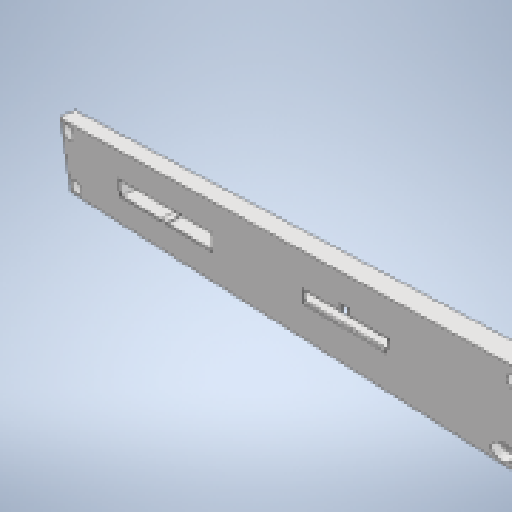
# Autodesk Inventor part: FrontPlate
Saved by Autodesk Inventor 2025.2 (Build 292293000, 293)
## iProperties
Created: 2025-08-10
Part Number: FrontPlate
Material: Generic
Document SubType Name: Modeling
Designer: hofma
Density: 1 g/cm^3
Appearance: Default
Author: hofma
Autodesk Inventor part; units mm, degrees
note: some values were not read from the file. Chosen so that the rebuilt part matches the saved one: direction of "Hole1".
ref_plane "YZ Plane" through (0, 0, 0) normal (1, 0, 0) x (0, 1, 0)
ref_plane "XZ Plane" through (0, 0, 0) normal (0, 1, 0) x (-1, 0, 0)
ref_plane "XY Plane" through (0, 0, 0) normal (0, 0, 1) x (1, 0, 0)
sketch "Sketch1" plane through (0, 0, 0) normal (0, 0, 1) x (1, 0, 0)
  line L0 (-125, 20) -> (125, 20)
  line L1 (125, 20) -> (125, -20)
  line L2 (125, -20) -> (-125, -20)
  line L3 (-125, -20) -> (-125, 20)
  line L4 (-125, 20) -> (125, -20) construction
  line L5 (125, 20) -> (-125, -20) construction
  point P0 (0, 0)
  dimension "d0" = 250
  dimension "d1" = 40
  constraints: 12 end point, 2 midpoint, 2 parallel, 1 horizontal, 1 perpendicular
  measures "d0" distance of L0.start L0.end
  measures "d1" distance of L2.end L0.start
extrude "Extrusion1" add sketch "Sketch1" along normal blind 10
sketch "Sketch2" plane through (0, 0, 10) normal (0, 0, 1) x (1, 0, 0)
  line L0 (30.75, 2.75) -> (69.25, 2.75)
  line L1 (69.25, 2.75) -> (69.25, -2.75)
  line L2 (69.25, -2.75) -> (30.75, -2.75)
  line L3 (30.75, -2.75) -> (30.75, 2.75)
  line L4 (-80.6, 4.125) -> (-19.4, 4.125)
  line L5 (-19.4, 4.125) -> (-19.4, -4.125)
  line L6 (-19.4, -4.125) -> (-80.6, -4.125)
  line L7 (-80.6, -4.125) -> (-80.6, 4.125)
  line L8 (-125, 20) -> (-125, -20) projected
  line L9 (-125, 0) -> (125, 0) construction
  line L10 (125, -20) -> (125, 20) projected
  line L11 (-125, 20) -> (0, 20) construction
  line L12 (125, 20) -> (-125, 20) construction
  line L13 (0, 20) -> (125, 20) construction
  line L14 (48.7, 2.75) -> (51.3, 2.75)
  line L15 (51.3, 2.75) -> (51.3, 5.95)
  line L16 (51.3, 5.95) -> (48.7, 5.95)
  line L17 (48.7, 5.95) -> (48.7, 2.75)
  point P0 (0, 0)
  point P1 (-62.5, 20)
  point P2 (-50, 4.125)
  point P3 (62.5, 20)
  point P4 (50, 2.75)
  point P5 (-19.4, 0)
  point P6 (30.75, 0)
  point P7 (50, 5.95)
  point P8 (0, 0)
  dimension "d5" = 61.2
  dimension "d6" = 8.25
  dimension "d7" = 0
  dimension "d8" = 38.5
  dimension "d9" = 5.5
  dimension "d10" = 2.6
  dimension "d12" = 8.7
  dimension "d35" = 50
  dimension "d52" = 50
  constraints: 30 end point, 11 midpoint, 6 parallel, 4 horizontal, 3 perpendicular, 3 point on line, 1 collinear, 1 vertical alignment
  measures "d5" distance of L4.start L4.end
  measures "d6" distance between parallel lines of L6 L4
  measures "d7" distance from line of point (0, 0) L9
  measures "d8" distance between parallel lines of L1 L3
  measures "d9" distance between parallel lines of L2 L0
  measures "d10" distance of L15.end L16.end
  measures "d12" distance between parallel lines of L16 L2
  measures "d35" horizontal distance of point (50, 5.95) point (0, 0)
  measures "d52" horizontal distance of point (0, 0) point (-50, 4.125)
extrude "Extrusion2" cut sketch "Sketch2" against normal through all
sketch "Sketch3" plane through (-80.6, -4.125, 10) normal (0, 1, 0) x (1, 0, 0)
  line L0 (0, 0) -> (0, 10) projected
  line L1 (61.2, 0) -> (61.2, 10) projected
  line L2 (-44.4, 0) -> (205.6, 0) projected
  line L3 (28.6, 0) -> (32.6, 0)
  line L4 (32.6, 0) -> (32.6, 7.6)
  line L5 (32.6, 7.6) -> (28.6, 7.6)
  line L6 (28.6, 7.6) -> (28.6, 0)
  line L7 (0, 10) -> (61.2, 10) construction
  line L8 (-44.4, 10) -> (205.6, 10) projected
  point P0 (80.6, 10)
  point P1 (30.6, 10)
  point P2 (30.6, 7.6)
  dimension "d15" = 4
  dimension "d16" = 7.6
  constraints: 10 end point, 2 midpoint, 2 parallel, 1 collinear, 1 horizontal, 1 perpendicular, 1 point on line, 1 vertical alignment
  measures "d15" distance of L4.end L5.end
  measures "d16" distance of L5.end L3.start
extrude "Extrusion3" add sketch "Sketch3" along normal blind 0.8 contours L6 L5 L4 L2
sketch "Sketch4" plane through (0, 0, 0) normal (0, 0, -1) x (-1, 0, 0)
  line L0 (-90, 5.95) -> (-10, 5.95)
  line L1 (-10, 5.95) -> (-10, -7.05)
  line L2 (-10, -7.05) -> (-90, -7.05)
  line L3 (-90, -7.05) -> (-90, 5.95)
  line L4 (-51.3, 5.95) -> (-48.7, 5.95) projected
  point P0 (0, 0)
  point P1 (-50, 5.95)
  point P2 (-50, 5.95)
  dimension "d19" = 80
  dimension "d20" = 13
  constraints: 8 end point, 3 midpoint, 2 parallel, 1 coincident, 1 horizontal, 1 perpendicular
  measures "d19" distance of L0.start L0.end
  measures "d20" distance of L2.end L0.start
extrude "Extrusion4" cut sketch "Sketch4" against normal blind 8
sketch "Sketch6" plane through (10, -7.05, 0) normal (0, 1, 0) x (1, 0, 0)
  line L0 (0, 0) -> (80, 0) projected
  line L1 (40, 0) -> (40, -18.0436) construction
  line L2 (-135, -10) -> (115, -10) projected
  line L3 (67.5, 0) -> (74.5, 0)
  line L4 (74.5, 0) -> (74.5, -10)
  line L5 (74.5, -10) -> (67.5, -10)
  line L6 (67.5, -10) -> (67.5, 0)
  line L7 (-135, 0) -> (115, 0) projected
  line L8 (5.5, -10) -> (12.5, -10)
  line L9 (12.5, -10) -> (12.5, 0)
  line L10 (12.5, 0) -> (5.5, 0)
  line L11 (5.5, 0) -> (5.5, -10)
  point P0 (-10, 0)
  point P1 (9, -10)
  point P2 (71, -10)
  dimension "d28" = 62
  dimension "d29" = 7
  constraints: 18 end point, 4 parallel, 3 midpoint, 3 point on line, 2 horizontal, 2 perpendicular, 1 vertical, 4 other
  measures "d28" distance of point (9, -10) point (71, -10)
  measures "d29" distance between parallel lines of L6 L4
extrude "Extrusion6" add sketch "Sketch6" along normal blind 3.116 contours L0 L9 L2 L11 | L0 L4 L2 L6
sketch "Sketch7" plane through (0, 0, 0) normal (0, 0, -1) x (-1, 0, 0)
  line L0 (-84.5, -3.934) -> (-77.5, -3.934) projected
  line L1 (-84.5, -7.05) -> (-84.5, -3.934) projected
  line L2 (-77.5, -7.05) -> (-77.5, -3.934) projected
  line L3 (-22.5, -3.934) -> (-15.5, -3.934) projected
  line L4 (-15.5, -7.05) -> (-15.5, -3.934) projected
  line L5 (-22.5, -7.05) -> (-22.5, -3.934) projected
  line L6 (-84.5, -7.05) -> (-90, -7.05) projected
  line L7 (-84.5, -7.05) -> (-77.5, -7.05)
  line L8 (-77.5, -7.05) -> (-77.5, -9.934)
  line L9 (-77.5, -9.934) -> (-84.5, -9.934)
  line L10 (-84.5, -9.934) -> (-84.5, -7.05)
  line L11 (-22.5, -7.05) -> (-77.5, -7.05) projected
  line L12 (-22.5, -7.05) -> (-15.5, -7.05)
  line L13 (-15.5, -7.05) -> (-15.5, -9.934)
  line L14 (-15.5, -9.934) -> (-22.5, -9.934)
  line L15 (-22.5, -9.934) -> (-22.5, -7.05)
  point P0 (0, 0)
  point P1 (-81, -9.934)
  point P2 (-19, -9.934)
  point P3 (-77.5, -5.492)
  point P4 (-77.5, -8.492)
  point P5 (-15.5, -5.492)
  point P6 (-15.5, -8.492)
  dimension "d32" = 6
  constraints: 16 end point, 6 midpoint, 4 parallel, 2 horizontal, 2 perpendicular, 2 vertical alignment, 1 horizontal alignment
  measures "d32" distance between parallel lines of L9 L0
extrude "Extrusion7" add sketch "Sketch7" along normal blind 2
sketch "Sketch8" plane through (0, 0, 10) normal (0, 0, 1) x (1, 0, 0)
  line L0 (125, 20) -> (-125, 20) projected
  line L1 (-125, 20) -> (-125, -20) projected
  line L2 (125, -20) -> (125, 20) projected
  line L3 (-125, -20) -> (125, -20) projected
  point P0 (0, 0)
  point P1 (-117.5, 15)
  point P2 (-117.5, -15)
  point P3 (117.5, 15)
  point P4 (117.5, -15)
  dimension "d36" = 5
  dimension "d37" = 7.5
  dimension "d38" = 7.5
  dimension "d39" = 5
  constraints: 2 horizontal alignment, 2 vertical alignment
  measures "d36" distance from line of point (-117.5, 15) L0
  measures "d37" distance from line of L1 point (-117.5, 15)
  measures "d38" distance from line of L2 point (117.5, 15)
  measures "d39" distance from line of L3 point (-117.5, -15)
hole "Hole1" at (117.5, -15, 10) at (-117.5, 15, 10) at (117.5, 15, 10) at (-117.5, -15, 10) direction (0, 0, -1) diameter 4.2 depth 10 counterbore diameter 8 counterbore depth 4.6 clearance for "Socket Head Cap Screw ISO 4762" size "M4" standard "ISO"
sketch "Sketch9" plane through (10, -3.934, 0) normal (0, 1, 0) x (1, 0, 0)
  circle A0 centre (71.05, -1.5002) radius 1.95 projected
  circle A1 centre (9.05, -1.5002) radius 1.95 projected
  point P0 (-10, 0)
extrude "Extrusion8" cut sketch "Sketch9" against normal blind 6
chamfer "Chamfer1" distance 7 angle 45 1 edges at (50, 5.95, 0)
chamfer "Chamfer2" distance 2 angle 45 2 edges at (-125, 0, 10) (125, 0, 10)
chamfer "Chamfer3" distance 0.5 angle 45 24 edges at (50, -2.75, 10) (30.75, 0, 10) (39.725, 2.75, 10) (48.7, 4.35, 10) (50, 5.95, 10) (51.3, 4.35, 10) (60.275, 2.75, 10) (69.25, 0, 10) (50, -2.75, 8) (69.25, 0, 8) (60.275, 2.75, 8) (51.3, 4.35, 8) (48.7, 4.35, 8) (39.725, 2.75, 8) (30.75, 0, 8) (-50, -4.125, 0) (-19.4, 0, 0) (-50, 4.125, 0) (-80.6, 0, 0) (-33.7, -4.125, 10) (-66.3, -4.125, 10) (-80.6, 0, 10) (-50, 4.125, 10) (-19.4, 0, 10)
fillet "Fillet1" radius 3.5 4 edges at (15.5, -6.934, -2) (22.5, -6.934, -2) (77.5, -6.934, -2) (84.5, -6.934, -2)
sketch "Sketch10" plane through (0, 0, 0) normal (0, 0, -1) x (-1, 0, 0)
  circle A0 centre (15, 0) radius 2
  circle A1 centre (85, 0) radius 2
  line L0 (18.9, 4.625) -> (81.1, 4.625) projected
  line L1 (50, 4.625) -> (50, 26.2106) construction
  line L2 (18.9, 4.625) -> (18.9, -4.625) projected
  point P0 (0, 0)
  point P1 (18.9, 0)
  dimension "d60" = 70
  dimension "d61" = 4
  constraints: 2 centre point, 2 end point, 2 midpoint, 1 horizontal alignment, 1 vertical, 1 other
  measures "d60" distance of A1.centre A0.centre
  measures "d61" diameter of A0
extrude "Extrusion9" cut sketch "Sketch10" against normal blind 5.7
equation "\"d38\" = d37"
equation "\"d39\" = d36"
body "Solid1"
